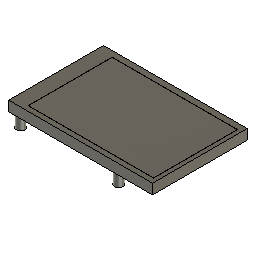
PolyPod (Autodesk Fusion 360 archive; units mm, degrees)
design "PolyPod_BottomScreen"
Autodesk Fusion 360 part; units mm, degrees
sketch "Sketch1" plane through (0, 0, 0) normal (0, 0, 1) x (1, 0, 0)
  line L0 (0, 0) -> (85, 0)
  line L1 (85, 0) -> (85, 56)
  line L2 (85, 56) -> (0, 56)
  line L3 (0, 56) -> (0, 0)
  dimension "d1" = 85
  dimension "d2" = 56
  constraint horizontal L0
  constraint vertical L1
  constraint horizontal L2
  constraint vertical L3
  constraint coincident L0.start L3.end
  measures "d1" distance of L0.start L0.end
  measures "d2" distance of L0.start L2.end
extrude "Extrude1" add sketch "Sketch1" along normal blind 6
sketch "Sketch2" plane through (0, 0, 6) normal (0, 0, 1) x (-1, 0, 0)
  line L0 (0, -56) -> (0, 0)
  line L1 (0, 0) -> (-85, 0)
  line L2 (-85, 0) -> (-85, -56)
  line L3 (-85, -56) -> (0, -56)
  line L4 (-85, 0) -> (-85, -3)
  line L5 (-85, -3) -> (-82.59, -3)
  line L6 (-82.59, -3) -> (-8.55, -3)
  line L7 (-8.55, -3) -> (-8.55, -52.56)
  line L8 (-8.55, -52.56) -> (-82.59, -52.56)
  line L9 (-82.59, -52.56) -> (-82.59, -3)
  dimension "d5" = 3
  dimension "d6" = 2.41
  dimension "d7" = 74.04
  dimension "d8" = 49.56
  constraint coincident L1.end L2.start
  constraint perpendicular L1 L4
  constraint perpendicular L4 L5
  constraint horizontal L6
  constraint vertical L7
  constraint horizontal L8
  constraint vertical L9
  measures "d5" distance of L1.end L4.end
  measures "d6" distance of L4.end L5.end
  measures "d7" distance of L5.end L6.end
  measures "d8" distance of L5.end L8.end
extrude "Extrude2" cut sketch "Sketch2" against normal blind 0.1 contours L6 L7 L8 L9
sketch "Sketch3" plane through (0, 0, 0) normal (0, 0, -1) x (1, 0, 0)
  line L0 (0, 0) -> (0, -56)
  line L1 (0, -56) -> (85, -56)
  line L2 (85, -56) -> (85, 0)
  line L3 (85, 0) -> (0, 0)
  line L4 (0, 0) -> (0, -56)
  circle A0 centre (3.48, -3.5) radius 1.25
  circle A1 centre (3.48, -52.5) radius 1.25
  circle A2 centre (3.48, -52.5) radius 2.5
  circle A3 centre (3.48, -3.5) radius 2.5
  circle A4 centre (61.48, -52.5) radius 1.25
  circle A5 centre (61.48, -3.5) radius 1.25
  circle A6 centre (61.48, -3.5) radius 2.5
  circle A7 centre (61.48, -52.5) radius 2.5
  dimension "d14" = 2.5
  dimension "d15" = 2.5
  dimension "d16" = 5
  dimension "d17" = 5
  dimension "d18" = 58
  dimension "d20" = 2.5
  dimension "d21" = 2.5
  dimension "d22" = 5
  dimension "d23" = 5
  constraint vertical L4
  constraint coincident L0.end L1.start
  constraint concentric A1 A2
  constraint concentric A0 A3
  constraint concentric A5 A6
  constraint concentric A4 A7
  measures "d14" diameter of A0
  measures "d15" diameter of A1
  measures "d16" diameter of A2
  measures "d17" diameter of A3
  measures "d18" distance of A0.centre A5.centre
  measures "d20" diameter of A4
  measures "d21" diameter of A5
  measures "d22" diameter of A6
  measures "d23" diameter of A7
extrude "Extrude3" add sketch "Sketch3" along normal blind 8 contours A2 | A3 | A6 | A7

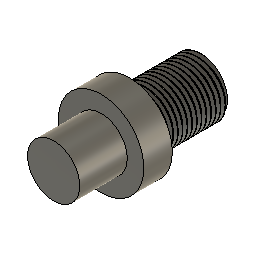
design "PolyPod_PowerConnection"
Autodesk Fusion 360 part; units mm, degrees
sketch "Sketch1" plane through (0, 0, 0) normal (0, 0, 1) x (1, 0, 0)
  line L0 (0, 0) -> (18, 0)
  line L1 (18, 0) -> (18, 6)
  line L2 (18, 6) -> (0, 6)
  line L3 (0, 6) -> (0, 0)
  line L4 (9, 6) -> (9, -14) construction
  line L5 (3.5, 0) -> (14.5, 0) construction
  line L6 (14.5, 0) -> (14.5, -10)
  line L7 (14.5, -10) -> (3.5, -10)
  line L8 (3.5, -10) -> (3.5, 0)
  line L9 (9, -10) -> (9, 0) construction
  line L10 (3.805, -10) -> (14.195, -10) construction
  line L11 (3.805, -10) -> (3.5, 0) construction
  line L12 (14.195, -10) -> (14.5, 0) construction
  line L13 (3.3, 6) -> (14.7, 6) construction
  line L14 (14.7, 6) -> (14.7, 21)
  line L15 (14.7, 21) -> (3.3, 21)
  line L16 (3.3, 21) -> (3.3, 6)
  line L17 (9, -10) -> (9, 21)
  point P0 (9, 0)
  point P1 (9, 6)
  dimension "d8" = 18
  dimension "d9" = 6
  dimension "d10" = 20
  dimension "d11" = 11
  dimension "d12" = 10
  dimension "d13" = 10.39
  dimension "d14" = 11.4
  dimension "d15" = 15
  constraint horizontal L0
  constraint vertical L1
  constraint horizontal L2
  constraint vertical L3
  constraint coincident L0.start L3.end
  constraint midpoint L2 P1
  constraint perpendicular L0 L4
  constraint horizontal L5
  constraint vertical L6
  constraint horizontal L7
  constraint vertical L8
  constraint coincident L0 L5.start
  constraint midpoint L0 P0
  constraint midpoint L7 L9.start
  constraint midpoint L5 P0
  constraint coincident P0 L9.end
  constraint midpoint L9.start L10
  constraint perpendicular L4 L10
  constraint horizontal L13
  constraint vertical L14
  constraint horizontal L15
  constraint vertical L16
  constraint midpoint L13 P1
  constraint coincident P1 L4.start
  constraint midpoint L15 L17.end
  measures "d8" distance of L0.start L0.end
  measures "d9" distance of L0.start L2.end
  measures "d10" distance of P1 L4.end
  measures "d11" distance of L5.start L5.end
  measures "d12" distance of L5.start L7.end
  measures "d13" distance of L10.start L10.end
  measures "d14" distance of L13.start L13.end
  measures "d15" distance of L13.start L15.end
revolve "Revolve1" add sketch "Sketch1" angle 360 about axis through (9, -10, 0) along (0, 1, 0) contours L0 L2 L3 L17 | L0 L7 L8 L17 | L2 L15 L16 L17
thread "Thread1" "ISO Metric profile 12.0 M12x1 M12x1 6g" major diameter 11.884 minor diameter 10.7405 pitch 1 angle 60 modelled right hand crest width 0.1426 on face at (3.3071, 11, -0.2841) crest through (3.058, 5.75, 0)
equation "InnerL = 10 mm"
equation "MidL = 6 mm"
equation "OuterL = 15 mm"
equation "InnerD = 11 mm" comment "Female side of usb c Diameter that meets to the midD"
equation "MidD = 18 mm"
equation "OuterD = 11.4 mm" comment "M12 threaded"
equation "InnerTaperD = 10.39 mm"
equation "d8 = MidD"
equation "d9 = MidL"
equation "d11 = InnerD"
equation "d12 = InnerL"
equation "d13 = InnerTaperD"
equation "d14 = OuterD"
equation "d15 = OuterL"

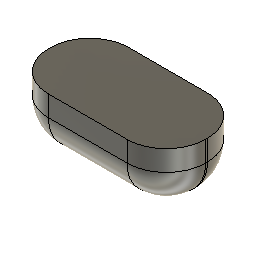
design "PolyPod_Speaker"
Autodesk Fusion 360 part; units mm, degrees
sketch "Sketch1" plane through (0, 0, 0) normal (0, 0, 1) x (1, 0, 0)
  line L0 (0, 0) -> (84, 0)
  line L1 (84, 0) -> (84, 43)
  line L2 (84, 43) -> (0, 43)
  line L3 (0, 43) -> (0, 0)
  dimension "d4" = 84
  dimension "d5" = 43
  constraint horizontal L0
  constraint vertical L1
  constraint horizontal L2
  constraint vertical L3
  constraint coincident L0.start L3.end
  measures "d4" distance of L0.start L0.end
  measures "d5" distance of L0.start L2.end
extrude "Extrude1" add sketch "Sketch1" along normal blind 32
fillet "Fillet1" radius 21 4 edges at (0, 0, 16) (0, 43, 16) (84, 43, 16) (84, 0, 16)
fillet "Fillet2" radius 21 8 edges at (0, 21.5, 0) (6.1508, 6.1508, 0) (42, 0, 0) (77.8492, 6.1508, 0) (84, 21.5, 0) (77.8492, 36.8492, 0) (42, 43, 0) (6.1508, 36.8492, 0)
equation "LSpeaker = 84 mm"
equation "WSpeaker = 43 mm"
equation "DSpeaker = 32 mm"
equation "d4 = LSpeaker"
equation "d5 = WSpeaker"
equation "d6 = DSpeaker"
